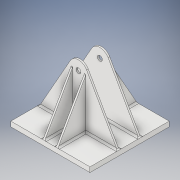
# Autodesk Inventor part: MM Base
Saved by Autodesk Inventor 2018 (Build 220112000, 112)
## iProperties
Created: 2018-02-19
Part Number: MM Base
Material: Iron, Malleable
Document SubType Name: Modeling
Designer: Marcus
Density: 7.15 g/cm^3
Appearance: White
Author: Marcus
Autodesk Inventor part; units mm, degrees
ref_plane "YZ Plane" through (0, 0, 0) normal (1, 0, 0) x (0, 1, 0)
ref_plane "XZ Plane" through (0, 0, 0) normal (0, 1, 0) x (-1, 0, 0)
sketch "Sketch1" plane through (0, 0, 0) normal (0, 1, 0) x (-1, 0, 0)
  line L0 (609.6, 609.6) -> (-609.6, 609.6)
  line L1 (-609.6, 609.6) -> (-609.6, -609.6)
  line L2 (-609.6, -609.6) -> (609.6, -609.6)
  line L3 (609.6, -609.6) -> (609.6, 609.6)
  line L4 (609.6, 609.6) -> (-609.6, -609.6) construction
  line L5 (-609.6, 609.6) -> (609.6, -609.6) construction
  point P0 (0, 0)
  dimension "d0" = 1219.2
  dimension "d1" = 1219.2
  constraints: 12 end point, 2 midpoint, 2 parallel, 1 horizontal, 1 perpendicular
  measures "d0" distance of L2.end L1.end
  measures "d1" distance of L1.end L0.end
extrude "Extrusion1" add sketch "Sketch1" along normal blind 76.2
ref_plane "Work Plane1" through (-609.6, 0, 0) normal (0, 0, 1) x (1, 0, 0)
sketch "Sketch2" plane through (-609.6, 0, 0) normal (0, 0, 1) x (1, 0, 0)
  line L0 (1219.2, 76.2) -> (0, 76.2) projected
  line L1 (12.7, 76.2) -> (483.3184, 909.5179)
  arc A0 (735.8816, 909.5179) -> (483.3184, 909.5179) centre (609.6, 838.2) ccw
  line L2 (735.8816, 909.5179) -> (1206.5, 76.2)
  line L3 (609.6, 76.2) -> (609.6, 838.2) construction
  point P0 (609.6, 0)
  dimension "d4" = 12.7
  dimension "d5" = 12.7
  dimension "d6" = 762
  constraints: 6 end point, 2 point on circle, 2 point on line, 2 tangent, 1 centre point, 1 midpoint, 1 vertical
  measures "d4" distance of L0.end L1.start
  measures "d5" distance of L0.start L2.end
  measures "d6" distance from line of L0 L3.end
extrude "Extrusion2" add sketch "Sketch2" along normal mid plane 355.6
hole "Hole1" at (0, 838.2, 177.8) direction (0, 0, -1) diameter 76.2 end through all
sketch "Sketch4" plane through (-609.6, 0, 609.6) normal (0, 0, 1) x (1, 0, 0)
  line L0 (0, 76.2) -> (1219.2, 76.2) construction
  circle A0 centre (609.6, 838.2) radius 38.1 construction
  line L1 (1206.5, 76.2) -> (12.7, 76.2) construction
  line L2 (1206.5, 76.2) -> (735.8816, 909.5179) construction
  arc A1 (735.8816, 909.5179) -> (483.3184, 909.5179) centre (609.6, 838.2) ccw construction
  line L3 (483.3184, 909.5179) -> (12.7, 76.2) construction
  line L4 (1206.5, 76.2) -> (12.7, 76.2) projected
  line L5 (520.7, 76.2) -> (495.3, 76.2)
  line L6 (495.3, 76.2) -> (495.3, 838.2)
  line L7 (495.3, 838.2) -> (520.7, 838.2)
  line L8 (520.7, 838.2) -> (520.7, 76.2)
  line L9 (698.5, 838.2) -> (723.9, 838.2)
  line L10 (723.9, 838.2) -> (723.9, 76.2)
  line L11 (723.9, 76.2) -> (698.5, 76.2)
  line L12 (698.5, 76.2) -> (698.5, 838.2)
  line L13 (776.1586, 838.2) -> (443.0414, 838.2) construction
  point P0 (609.6, 0)
  dimension "d23" = 177.8
  dimension "d24" = 25.4
  dimension "d25" = 88.9
  constraints: 18 end point, 5 point on line, 4 parallel, 3 horizontal, 2 collinear, 2 perpendicular, 1 coincident, 1 midpoint
  measures "d23" distance between parallel lines of L12 L8
  measures "d24" distance between parallel lines of L8 L6
  measures "d25" distance from line of A0.centre L12
extrude "Extrusion4" add sketch "Sketch4" against normal up to surface (1219.2 mm away)
sketch "Sketch5" plane through (609.6, 0, 609.6) normal (1, 0, 0) x (0, 0, -1)
  line L0 (0, 76.2) -> (1219.2, 76.2) construction
  line L1 (431.8, 76.2) -> (431.8, 909.5179) construction
  line L2 (431.8, 983.2286) -> (431.8, 909.5179) projected
  line L3 (787.4, 983.2286) -> (431.8, 983.2286) projected
  line L4 (787.4, 909.5179) -> (787.4, 909.5179) projected
  line L5 (787.4, 909.5179) -> (787.4, 76.2) construction
  line L6 (457.2, 76.2) -> (457.2, 983.2286)
  line L7 (762, 983.2286) -> (762, 76.2)
  line L8 (762, 76.2) -> (457.2, 76.2)
  line L9 (457.2, 983.2286) -> (762, 983.2286)
  line L10 (0, 76.2) -> (0, 838.2) construction
  line L11 (0, 838.2) -> (431.8, 838.2) construction
  line L12 (787.4, 838.2) -> (1219.2, 838.2) construction
  line L13 (1219.2, 76.2) -> (1219.2, 838.2) construction
  line L14 (0, 76.2) -> (431.8, 838.2)
  line L15 (431.8, 838.2) -> (0, 838.2)
  line L16 (0, 0) -> (0, 76.2) projected
  line L17 (0, 838.2) -> (0, 76.2)
  line L18 (1219.2, 76.2) -> (0, 76.2) projected
  line L19 (787.4, 838.2) -> (1219.2, 76.2)
  line L20 (1219.2, 838.2) -> (1219.2, 76.2) projected
  line L21 (1219.2, 76.2) -> (1219.2, 838.2)
  line L22 (1219.2, 838.2) -> (787.4, 838.2)
  point P0 (609.6, 0)
  dimension "d28" = 25.4
  dimension "d29" = 25.4
  constraints: 20 end point, 5 perpendicular, 4 point on line, 2 collinear, 1 horizontal, 1 vertical alignment
  measures "d28" distance between parallel lines of L1 L6
  measures "d29" distance between parallel lines of L5 L7
extrude "Extrusion6" cut sketch "Sketch5" against normal through all
fillet "Fillet1" radius 25.4 8 edges at (101.6, 838.2, 177.8) (-101.6, 838.2, 177.8) (101.6, 838.2, -177.8) (-101.6, 838.2, -177.8) (596.9, 76.2, -165.1) (596.9, 76.2, 165.1) (-596.9, 76.2, -165.1) (-596.9, 76.2, 165.1)
fillet "Fillet2" radius 25.4 16 edges at (114.3, 76.2, 393.7) (-88.9, 76.2, 393.7) (88.9, 76.2, 393.7) (-114.3, 76.2, 393.7) (361.95, 76.2, 177.8) (0, 76.2, 152.4) (-361.95, 76.2, 177.8) (0, 76.2, -152.4) (361.95, 76.2, -177.8) (-361.95, 76.2, -177.8) (114.3, 76.2, -393.7) (88.9, 76.2, -393.7) (-88.9, 76.2, -393.7) (-114.3, 76.2, -393.7) (0, 76.2, 177.8) (0, 76.2, -177.8)
body "Solid1"
